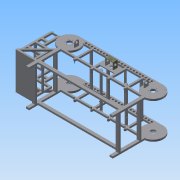
# Autodesk Inventor part: 整体支架
Saved by Autodesk Inventor 2015 (Build 190159000, 159)
## iProperties
Created: 2017-05-04
Part Number: 整体支架
Material: 常规
Document SubType Name: Modeling
Designer: Administrator
Density: 1 g/cm^3
Appearance: 默认
Author: Administrator
Autodesk Inventor part; units mm, degrees
ref_plane "YZ Plane" through (0, 0, 0) normal (1, 0, 0) x (0, 1, 0)
ref_plane "XZ Plane" through (0, 0, 0) normal (0, 1, 0) x (-1, 0, 0)
sketch "草图1" plane through (0, 0, 0) normal (0, 0, 1) x (1, 0, 0)
  circle A0 centre (0, 0) radius 141.3842
  line L0 (-50, 166.3842) -> (50, 166.3842)
  line L1 (50, 166.3842) -> (50, 141.3842)
  line L2 (50, 141.3842) -> (-50, 141.3842)
  line L3 (-50, 141.3842) -> (-50, 166.3842)
  line L4 (0, 0) -> (0, 76.7752)
  line L5 (0, 0) -> (71.7187, 0)
  line L6 (-57.3473, 163.9969) -> (-42.6527, 143.7715)
  line L7 (-42.6527, 143.7715) -> (-123.5544, 84.9929)
  line L8 (-123.5544, 84.9929) -> (-138.249, 105.2184)
  line L9 (-142.7899, 98.9684) -> (-119.0135, 91.2429)
  line L10 (-119.0135, 91.2429) -> (-149.9152, -3.8627)
  line L11 (-149.9152, -3.8627) -> (-173.6916, 3.8627)
  line L12 (-173.6916, -3.8627) -> (-149.9152, 3.8627)
  line L13 (-149.9152, 3.8627) -> (-119.0135, -91.2429)
  line L14 (-119.0135, -91.2429) -> (-142.7899, -98.9684)
  line L15 (-138.249, -105.2184) -> (-123.5544, -84.9929)
  line L16 (-123.5544, -84.9929) -> (-42.6527, -143.7715)
  line L17 (-42.6527, -143.7715) -> (-57.3473, -163.9969)
  line L18 (-50, -166.3842) -> (-50, -141.3842)
  line L19 (-50, -141.3842) -> (50, -141.3842)
  line L20 (50, -141.3842) -> (50, -166.3842)
  line L21 (-10, 166.3842) -> (-20, 141.3842)
  line L22 (10, 166.3842) -> (20, 141.3842)
  arc A1 (18.4913, 145.1558) -> (24.0622, 141.3842) centre (24.0622, 147.3842) ccw
  arc A2 (-24.0622, 141.3842) -> (-18.4913, 145.1558) centre (-24.0622, 147.3842) ccw
  arc A3 (-19.7673, 141.9659) -> (-40.4509, 137.5092) centre (0, 0) ccw
  circle A4 centre (150, 128.8842) radius 12.5
  circle A5 centre (150, 128.8842) radius 17.5
  line L23 (0, 168.8842) -> (1400, 168.8842)
  line L24 (1400, 168.8842) -> (1400, 101.3842)
  line L25 (1400, 101.3842) -> (0, 101.3842)
  line L26 (0, 101.3842) -> (0, 168.8842)
  circle A6 centre (200, 128.8842) radius 17.5
  circle A7 centre (250, 128.8842) radius 17.5
  circle A8 centre (300, 128.8842) radius 17.5
  circle A9 centre (350, 128.8842) radius 17.5
  circle A10 centre (400, 128.8842) radius 17.5
  circle A11 centre (450, 128.8842) radius 17.5
  circle A12 centre (500, 128.8842) radius 17.5
  circle A13 centre (550, 128.8842) radius 17.5
  circle A14 centre (600, 128.8842) radius 17.5
  circle A15 centre (650, 128.8842) radius 17.5
  circle A16 centre (700, 128.8842) radius 17.5
  circle A17 centre (750, 128.8842) radius 17.5
  circle A18 centre (800, 128.8842) radius 17.5
  circle A19 centre (850, 128.8842) radius 17.5
  circle A20 centre (900, 128.8842) radius 17.5
  circle A21 centre (950, 128.8842) radius 17.5
  circle A22 centre (1000, 128.8842) radius 17.5
  circle A23 centre (1050, 128.8842) radius 17.5
  circle A24 centre (1100, 128.8842) radius 17.5
  circle A25 centre (1150, 128.8842) radius 17.5
  circle A26 centre (1200, 128.8842) radius 17.5
  circle A27 centre (1250, 128.8842) radius 17.5
  line L27 (265, 101.3842) -> (295, 101.3842)
  line L28 (295, 101.3842) -> (295, -191.3842)
  line L29 (265, -191.3842) -> (265, 101.3842)
  arc A28 (280, -166.3842) -> (265, -171.3842) centre (280, -191.3842) ccw
  line L30 (0, -166.3842) -> (1400, -166.3842)
  line L31 (1400, -166.3842) -> (1400, -141.3842)
  line L32 (1400, -141.3842) -> (0, -141.3842)
  line L33 (0, -141.3842) -> (0, -166.3842)
  arc A29 (265, -191.3842) -> (295, -191.3842) centre (280, -191.3842) ccw
  line L34 (545, 101.3842) -> (575, 101.3842)
  line L35 (575, 101.3842) -> (575, -191.3842)
  line L36 (545, -191.3842) -> (545, 101.3842)
  arc A30 (545, -191.3842) -> (575, -191.3842) centre (560, -191.3842) ccw
  line L37 (825, 101.3842) -> (855, 101.3842)
  line L38 (855, 101.3842) -> (855, -191.3842)
  line L39 (825, -191.3842) -> (825, 101.3842)
  arc A31 (825, -191.3842) -> (855, -191.3842) centre (840, -191.3842) ccw
  line L40 (1105, 101.3842) -> (1135, 101.3842)
  line L41 (1135, 101.3842) -> (1135, -191.3842)
  line L42 (1105, -191.3842) -> (1105, 101.3842)
  arc A32 (1105, -191.3842) -> (1135, -191.3842) centre (1120, -191.3842) ccw
  point P0 (0, 166.3842)
  point P1 (-50, 153.8842)
  point P2 (545, -171.3842)
  point P3 (825, -171.3842)
  point P4 (1105, -171.3842)
  dimension "d0" = 76.7752
  dimension "d1" = 71.7187
  dimension "d2" = 25
  dimension "d3" = 100
  dimension "d6" = 180
  dimension "d8" = 20
  dimension "d9" = 40
  dimension "d11" = 12
  dimension "d12" = 12
  dimension "d13" = 20.6835
  dimension "d14" = 25
  dimension "d15" = 35
  dimension "d16" = 150
  dimension "d17" = 40
  dimension "d18" = 27.5
  dimension "d19" = 1400
  dimension "d22" = 50
  dimension "d27" = 30
  dimension "d28" = 265
  dimension "d29" = 50
  dimension "d32" = 1400
  dimension "d33" = 25
  dimension "d36" = 280
  constraints: 86 end point, 33 centre point, 17 point on line, 16 point on circle, 10 tangent, 7 horizontal, 7 parallel, 4 perpendicular, 3 coincident, 3 midpoint, 2 collinear, 2 concentric, 1 vertical, 111 other
  measures "d0" distance of L4.start L4.end
  measures "d1" distance of L4.start L5.end
  measures "d2" distance of L2.end L0.start
  measures "d3" distance of L0.start L0.end
  measures "d8" distance of L22.start L21.start
  measures "d9" distance of L22.end L21.end
  measures "d11" diameter of A1
  measures "d12" diameter of A2
  measures "d13" horizontal distance of A3.start A3.end
  measures "d14" diameter of A4
  measures "d15" diameter of A5
  measures "d16" distance from line of L4 A4.centre
  measures "d17" distance from line of L23 A5.centre
  measures "d18" distance from line of L25 A4.centre
  measures "d19" distance of L23.start L23.end
  measures "d22" distance of A5.centre A6.centre
  measures "d27" distance between parallel lines of L28 L29
  measures "d28" distance from line of point (0, 0) L29
  measures "d29" diameter of A28
  measures "d32" distance of L32.end L31.end
  measures "d33" distance of L32.end L30.start
  measures "d36" distance of L29.start L36.start
extrude "拉伸1" add sketch "草图1" against normal blind 30 contours L19 L20 L30 L33 | L32 L29 L30 L20 | L25 L26 A0 | A0 L2 L1 L0 L26 L23 L24 L25 | L32 L28 L30 L29 | L29 L25 L28 L32 | L26 L0 L22 L2 | L30 A28 L29 | L32 L36 L30 L28 | A28 L30 L28 A29 L29 | L36 L25 L35 L32 | L32 L35 L30 L36 | A1 L22 L0 L1 L2 | L30 L35 A30 L36 | L32 L39 L30 L35 | L39 L25 L38 L32 | L32 L38 L30 L39 | L30 L38 A31 L39 | L32 L42 L30 L38 | L41 L32 L42 L25 | L32 L41 L30 L42 | L32 L31 L30 L41 | L30 L41 A32 L42 picked at (61.7806, 104.7908)
sketch "草图2" plane through (0, 0, 0) normal (0, 0, 1) x (1, 0, 0)
  circle A0 centre (0, 0) radius 168.8842
  line L0 (1400, 168.8842) -> (0, 168.8842) projected
  line L1 (0, -166.3842) -> (1400, -166.3842)
  line L2 (1400, -166.3842) -> (1400, -168.8842)
  line L3 (1400, -168.8842) -> (0, -168.8842)
  line L4 (0, -168.8842) -> (0, -166.3842)
  circle A1 centre (1400, 0) radius 168.8842
  dimension "d45" = 1400
  constraints: 8 end point, 2 centre point, 2 horizontal, 2 parallel, 2 tangent, 1 coincident, 1 perpendicular, 2 other
  measures "d45" distance of A0.centre A1.centre
extrude "拉伸2" add sketch "草图2" against normal blind 30 contours A0 L1 L4 | L1 A1 L3 A0 | A0 L4 L1 | A1 L2 L1 | L1 L2 A1
sketch "草图5" plane through (0, 0, 0) normal (0, 0, 1) x (1, 0, 0)
  line L0 (-25, -167.0235) -> (25, -167.0235)
  line L1 (25, -167.0235) -> (25, -700)
  line L2 (25, -700) -> (-25, -700)
  line L3 (-25, -700) -> (-25, -167.0235)
  arc A0 (0, 168.8842) -> (0, -168.8842) centre (0, 0) ccw projected
  dimension "d67" = 700
  dimension "d68" = 50
  constraints: 8 end point, 2 parallel, 2 point on circle, 1 horizontal, 1 perpendicular
  measures "d67" distance from line of point (0, 0) L2
  measures "d68" distance of L1.end L2.end
extrude "拉伸5" add sketch "草图5" against normal blind 30
pattern_linear "矩形阵列2" count 2 spacing 1400 along (1, 0, 0) of "拉伸5"
sketch "草图6" plane through (0, 0, 0) normal (0, 0, 1) x (1, 0, 0)
  line L0 (25, -168.8842) -> (25, -700) projected
  line L1 (1375, -700) -> (1375, -168.8842) projected
  line L2 (25, -500) -> (1375, -500)
  line L3 (1375, -500) -> (1375, -550)
  line L4 (1375, -550) -> (25, -550)
  line L5 (25, -550) -> (25, -500)
  point P0 (0, 0)
  dimension "d74" = 500
  dimension "d75" = 50
  constraints: 8 end point, 2 parallel, 2 point on line, 1 horizontal, 1 perpendicular
  measures "d74" distance from line of point (0, 0) L2
  measures "d75" distance between parallel lines of L2 L4
extrude "拉伸6" add sketch "草图6" against normal blind 30
pattern_linear "矩形阵列14" count 2 spacing 590 along (0, 0, -1) of "拉伸1", "拉伸6", "拉伸5", "矩形阵列2", "拉伸2"
sketch "草图9" plane through (-25, -700, -590) normal (-1, 0, 0) x (0, 0, 1)
  line L0 (-30, 100) -> (590, 100)
  line L1 (590, 100) -> (590, 130)
  line L2 (590, 130) -> (-30, 130)
  line L3 (-30, 130) -> (-30, 100)
  line L4 (-30, 0) -> (-30, 532.9765) projected
  line L5 (590, 0) -> (590, 532.9765) projected
  line L6 (0, 0) -> (-30, 0) projected
  point P0 (590, 700)
  dimension "d138" = 30
  dimension "d139" = 100
  constraints: 8 end point, 2 collinear, 2 parallel, 1 horizontal, 1 perpendicular
  measures "d138" distance of L2.end L0.start
  measures "d139" distance between parallel lines of L6 L0
extrude "拉伸9" add sketch "草图9" against normal blind 50
pattern_linear "矩形阵列15" count 2 spacing 1400 along (1, 0, 0) of "拉伸9"
sketch "草图10" plane through (0, 0, 0) normal (0, 0, 1) x (1, 0, 0)
  line L0 (295, -141.3842) -> (295, 101.3842) projected
  line L1 (265, 101.3842) -> (295, 101.3842)
  line L2 (295, 101.3842) -> (295, 71.3842)
  line L3 (295, 71.3842) -> (265, 71.3842)
  line L4 (265, 71.3842) -> (265, 101.3842)
  point P0 (0, 0)
  dimension "d145" = 30
  constraints: 8 end point, 2 parallel, 1 horizontal, 1 perpendicular, 1 point on line
  measures "d145" distance between parallel lines of L1 L3
extrude "拉伸10" add sketch "草图10" against normal blind 590
pattern_linear "矩形阵列16" count 4 spacing 280 along (1, 0, 0) of "拉伸10"
pattern_linear "矩形阵列17" count 2 spacing 350 along (0, 1, 0) of "拉伸9", "矩形阵列15"
sketch "草图11" plane through (0, 0, 0) normal (0, 0, 1) x (1, 0, 0)
  circle A0 centre (1400, 0) radius 40
  arc A1 (1264.9329, 101.3842) -> (1307.6291, -141.3842) centre (1400, 0) ccw projected
  point P0 (0, 0)
  dimension "d154" = 80
  constraints: 1 centre point, 1 concentric
  measures "d154" diameter of A0
extrude "拉伸11" cut sketch "草图11" against normal blind 30
sketch "草图12" plane through (0, 0, 0) normal (0, 0, 1) x (1, 0, 0)
  circle A0 centre (1400, 55) radius 4
  circle A1 centre (1400, 0) radius 40
  circle A2 centre (1400, 0) radius 40 projected
  line L0 (1400, 0) -> (1400, 25)
  point P0 (0, 0)
  dimension "d157" = 80
  dimension "d158" = 25
  dimension "d159" = 55
  dimension "d160" = 8
  constraints: 2 centre point, 2 end point, 1 concentric, 1 point on line, 1 vertical
  measures "d157" diameter of A1
  measures "d158" distance of L0.start L0.end
  measures "d159" distance of A1.centre A0.centre
  measures "d160" diameter of A0
extrude "拉伸12" cut sketch "草图12" against normal blind 30 contours A0
thread "螺纹5" size "M8x1.25" class "6H" standard "ANSI Metric M Profile" full length
pattern_circular "环形阵列3" count 6 over 360 about axis through (1400, 0, 0) along (0, 0, -1) of "拉伸12"
sketch "草图13" plane through (0, 168.8842, -590) normal (0, 0, 1) x (1, 0, 0)
  circle A0 centre (1400, -168.8842) radius 40
  circle A1 centre (1400, -168.8842) radius 40 projected
  point P0 (0, -168.8842)
  dimension "d168" = 80
  constraints: 1 centre point, 1 concentric
  measures "d168" diameter of A0
extrude "拉伸13" cut sketch "草图13" against normal blind 18
sketch "草图14" plane through (1400, 0, -608) normal (0, 0, 1) x (1, 0, 0)
  circle A0 centre (0, 0) radius 31
  circle A1 centre (0, 0) radius 40 projected
  point P0 (-1400, 0)
  dimension "d171" = 62
  constraints: 1 centre point, 1 concentric
  measures "d171" diameter of A0
extrude "拉伸14" cut sketch "草图14" against normal blind 5 contours A0
sketch "草图15" plane through (1400, 0, -613) normal (0, 0, 1) x (1, 0, 0)
  circle A0 centre (0, 0) radius 20
  circle A1 centre (0, 0) radius 31 projected
  point P0 (-1400, 0)
  dimension "d174" = 40
  constraints: 1 centre point, 1 concentric
  measures "d174" diameter of A0
extrude "拉伸15" cut sketch "草图15" against normal through all contours A0
pattern_linear "矩形阵列18" count 2 spacing 1400 along (-1, 0, 0) of "拉伸11", "拉伸12", "环形阵列3", "拉伸13", "拉伸14", "拉伸15"
sketch "草图16" plane through (0, 0, 0) normal (0, 0, 1) x (1, 0, 0)
  circle A0 centre (127.5, 151.3842) radius 2
  circle A1 centre (127.5, 106.3842) radius 2
  circle A2 centre (150, 128.8842) radius 17.5 projected
  point P0 (0, 0)
  dimension "d180" = 4
  dimension "d181" = 4
  dimension "d182" = 22.5
  dimension "d183" = 22.5
  dimension "d184" = 22.5
  dimension "d185" = 22.5
  constraints: 2 centre point
  measures "d180" diameter of A0
  measures "d181" diameter of A1
  measures "d182" horizontal distance of A2.centre A0.centre
  measures "d183" horizontal distance of A2.centre A1.centre
  measures "d184" horizontal distance of A2.centre A0.centre
  measures "d185" horizontal distance of A2.centre A1.centre
extrude "拉伸16" cut sketch "草图16" against normal through all contours A0 | A1
thread "螺纹6" size "M4x0.7" class "6H" standard "ANSI Metric M Profile" full length
thread "螺纹7" size "M4x0.7" class "6H" standard "ANSI Metric M Profile" full length
thread "螺纹8" size "M4x0.7" class "6H" standard "ANSI Metric M Profile" full length
thread "螺纹9" size "M4x0.7" class "6H" standard "ANSI Metric M Profile" full length
pattern_linear "矩形阵列19" count 2 spacing 1145 along (1, 0, 0) of "拉伸16"
pattern_linear "矩形阵列20" count 2 spacing 197.5 along (1, 0, 0) of "拉伸16"
pattern_linear "矩形阵列21" count 6 spacing 150 along (1, 0, 0) of "矩形阵列20"
sketch "草图17" plane through (0, 0, -30) normal (0, 0, -1) x (-1, 0, 0)
  circle A0 centre (-280, -191.3842) radius 10
  arc A1 (-295, -191.3842) -> (-265, -191.3842) centre (-280, -191.3842) ccw projected
  point P0 (0, 0)
  dimension "d205" = 20
  constraints: 1 centre point, 1 concentric
  measures "d205" diameter of A0
extrude "拉伸17" add sketch "草图17" along normal blind 5
sketch "草图18" plane through (280, -191.3842, -35) normal (0, 0, -1) x (-1, 0, 0)
  circle A0 centre (0, 0) radius 5
  circle A1 centre (0, 0) radius 10 projected
  point P0 (280, 191.3842)
  dimension "d208" = 10
  constraints: 1 centre point, 1 concentric
  measures "d208" diameter of A0
extrude "拉伸18" add sketch "草图18" along normal blind 28 contours A0
thread "螺纹10" size "M10x1.5" class "6g" standard "ANSI Metric M Profile" length 10
chamfer "倒角1" distance 0.25 angle 45 1 edges at (285, -191.3842, -63)
ref_plane "工作平面1" through (0, 0, -310) normal (0, 0, -1) x (-1, 0, 0)
mirror "镜像1" about plane through (0, 0, -310) normal (0, 0, -1) of "拉伸17", "拉伸18", "倒角1"
pattern_linear "矩形阵列22" count 4 spacing 280 along (1, 0, 0) of "拉伸17", "拉伸18", "倒角1", "镜像1"
sketch "草图19" plane through (0, 0, 0) normal (0, 0, 1) x (1, 0, 0)
  circle A0 centre (1410, 152.6729) radius 2.5
  arc A1 (1422.9168, 151.274) -> (1410, 152.6729) centre (1400, 0) ccw
  circle A2 centre (1400, 0) radius 40 projected
  point P0 (0, 0)
  dimension "d219" = 5
  dimension "d220" = 153
  dimension "d221" = 10
  constraints: 2 centre point, 2 point on circle, 1 concentric
  measures "d219" diameter of A0
  measures "d220" radius of A1
  measures "d221" horizontal distance of A1.centre A0.centre
extrude "拉伸19" cut sketch "草图19" against normal through all contours A0
thread "螺纹11" size "M5x0.8" class "6H" standard "ANSI Metric M Profile" full length
thread "螺纹12" size "M5x0.8" class "6H" standard "ANSI Metric M Profile" full length
pattern_circular "环形阵列4" count 6 over 172.5 about axis through (1400, 0, 0) along (0, 0, -1) of "拉伸19"
sketch "草图20" plane through (0, 168.8842, 0) normal (0, 1, 0) x (1, 0, 0)
  circle A0 centre (1390, 11) radius 4
  line L0 (1400, 0) -> (0, 0) projected
  line L1 (1400, 0) -> (1400, 30) projected
  circle A1 centre (1390, 609) radius 4
  line L2 (0, 620) -> (1400, 620) projected
  line L3 (1400, 590) -> (1400, 620) projected
  dimension "d231" = 8
  dimension "d232" = 11
  dimension "d233" = 10
  dimension "d234" = 8
  dimension "d235" = 11
  dimension "d236" = 10
  constraints: 2 centre point
  measures "d231" diameter of A0
  measures "d232" distance from line of L0 A0.centre
  measures "d233" distance from line of L1 A0.centre
  measures "d234" diameter of A1
  measures "d235" distance from line of L2 A1.centre
  measures "d236" distance from line of L3 A1.centre
extrude "拉伸20" cut sketch "草图20" against normal blind 22
thread "螺纹13" size "M8x1.25" class "6H" standard "ANSI Metric M Profile" full length
thread "螺纹14" size "M8x1.25" class "6H" standard "ANSI Metric M Profile" full length
pattern_linear "矩形阵列23" count 5 spacing 220 along (-1, 0, 0) of "拉伸20"
sketch "草图21" plane through (0, 168.8842, 0) normal (0, 1, 0) x (1, 0, 0)
  circle A0 centre (20, 13) radius 4
  circle A1 centre (113.75, 13) radius 4
  circle A2 centre (207.5, 13) radius 4
  circle A3 centre (20, 607) radius 4
  line L0 (135.0671, 590) -> (135.0671, 620) projected
  line L1 (265, 590) -> (92.3709, 590) projected
  circle A4 centre (113.75, 607) radius 4
  line L2 (0, 590) -> (0, 620) projected
  line L3 (0, 620) -> (1400, 620) projected
  circle A5 centre (207.5, 607) radius 4
  line L4 (0, 0) -> (0, 30) projected
  line L5 (1400, 0) -> (0, 0) projected
  dimension "d246" = 8
  dimension "d247" = 8
  dimension "d248" = 8
  dimension "d249" = 8
  dimension "d252" = 8
  dimension "d253" = 20
  dimension "d254" = 13
  dimension "d255" = 13
  dimension "d256" = 113.75
  dimension "d257" = 8
  dimension "d258" = 13
  dimension "d259" = 207.5
  dimension "d260" = 20
  dimension "d261" = 13
  dimension "d262" = 113.75
  dimension "d263" = 207.5
  dimension "d264" = 13
  dimension "d265" = 13
  constraints: 6 centre point
  measures "d246" diameter of A0
  measures "d247" diameter of A1
  measures "d248" diameter of A2
  measures "d249" diameter of A3
  measures "d252" diameter of A4
  measures "d253" distance from line of L2 A3.centre
  measures "d254" distance from line of L3 A3.centre
  measures "d255" distance from line of L3 A4.centre
  measures "d256" distance from line of L2 A4.centre
  measures "d257" diameter of A5
  measures "d258" distance from line of A5.centre L3
  measures "d259" distance from line of L2 A5.centre
  measures "d260" distance from line of L4 A0.centre
  measures "d261" distance from line of L5 A0.centre
  measures "d262" distance from line of L4 A1.centre
  measures "d263" distance from line of L4 A2.centre
  measures "d264" distance from line of L5 A1.centre
  measures "d265" distance from line of L5 A2.centre
extrude "拉伸21" cut sketch "草图21" against normal blind 22
thread "螺纹15" size "M8x1.25" class "6H" standard "ANSI Metric M Profile" full length
thread "螺纹16" size "M8x1.25" class "6H" standard "ANSI Metric M Profile" full length
thread "螺纹17" size "M8x1.25" class "6H" standard "ANSI Metric M Profile" full length
thread "螺纹18" size "M8x1.25" class "6H" standard "ANSI Metric M Profile" full length
thread "螺纹19" size "M8x1.25" class "6H" standard "ANSI Metric M Profile" full length
thread "螺纹20" size "M8x1.25" class "6H" standard "ANSI Metric M Profile" full length
sketch "草图22" plane through (0, 0, 0) normal (0, 0, 1) x (1, 0, 0)
  line L0 (-25, -570) -> (-25, -250) projected
  line L1 (-25, -550) -> (-350, -550)
  line L2 (-350, -550) -> (-350, -520)
  line L3 (-350, -520) -> (-25, -520)
  line L4 (-25, -520) -> (-25, -550)
  line L5 (25, -500) -> (1375, -500) projected
  line L6 (1375, -550) -> (25, -550) projected
  point P0 (0, 0)
  dimension "d280" = 325
  dimension "d281" = 30
  constraints: 8 end point, 2 parallel, 1 collinear, 1 horizontal, 1 perpendicular, 1 point on line
  measures "d280" distance of L1.start L1.end
  measures "d281" distance of L1.end L2.end
extrude "拉伸22" add sketch "草图22" against normal up to surface (620 mm away)
sketch "草图23" plane through (0, 0, 0) normal (0, 0, 1) x (1, 0, 0)
  line L0 (-350, -520) -> (-25, -195)
  line L1 (-25, -520) -> (-25, -167.0235) projected
  line L2 (-307.5736, -520) -> (-25, -237.4264)
  line L3 (-25, -520) -> (-350, -520) projected
  line L4 (-350, -520) -> (-25, -520) projected
  line L5 (-350, -520) -> (-307.5736, -520)
  line L6 (-25, -195) -> (-25, -237.4264)
  point P0 (0, 0)
  dimension "d284" = 135
  dimension "d285" = 30
  constraints: 8 end point, 5 point on line, 1 collinear, 1 parallel
  measures "d284" angle of L3 L2
  measures "d285" distance between parallel lines of L0 L2
extrude "拉伸23" add sketch "草图23" against normal blind 30 contours L0 L1 L2 L3
pattern_linear "矩形阵列24" count 2 spacing 590 along (0, 0, -1) of "拉伸23"
sketch "草图25" plane through (0, 168.8842, -590) normal (0, 0, 1) x (1, 0, 0)
  line L0 (-350, -688.8842) -> (-70, -688.8842)
  line L1 (-70, -688.8842) -> (-70, -388.8842)
  line L2 (-70, -388.8842) -> (-350, -388.8842)
  line L3 (-350, -388.8842) -> (-350, -688.8842)
  line L4 (-200, -388.8842) -> (-350, -388.8842)
  line L5 (-350, -388.8842) -> (-350, -108.8842)
  line L6 (-350, -108.8842) -> (-200, -108.8842)
  line L7 (-200, -108.8842) -> (-200, -388.8842)
  line L8 (-320, -418.8842) -> (-100, -418.8842)
  line L9 (-100, -418.8842) -> (-100, -523.8842)
  line L10 (-100, -523.8842) -> (-320, -523.8842)
  line L11 (-320, -523.8842) -> (-320, -418.8842)
  line L12 (-320, -553.8842) -> (-100, -553.8842)
  line L13 (-100, -553.8842) -> (-100, -658.8842)
  line L14 (-100, -658.8842) -> (-320, -658.8842)
  line L15 (-320, -658.8842) -> (-320, -553.8842)
  line L16 (-320, -138.8842) -> (-230, -138.8842)
  line L17 (-230, -138.8842) -> (-230, -288.8842)
  line L18 (-230, -288.8842) -> (-320, -288.8842)
  line L19 (-320, -288.8842) -> (-320, -138.8842)
  line L20 (-320, -318.8842) -> (-230, -318.8842)
  line L21 (-230, -318.8842) -> (-230, -388.8842)
  line L22 (-230, -388.8842) -> (-320, -388.8842)
  line L23 (-320, -388.8842) -> (-320, -318.8842)
  point P0 (0, -168.8842)
  dimension "d291" = 280
  dimension "d292" = 300
  dimension "d293" = 150
  dimension "d294" = 280
  dimension "d295" = 30
  dimension "d296" = 30
  dimension "d297" = 30
  dimension "d298" = 30
  dimension "d299" = 30
  dimension "d300" = 30
  dimension "d301" = 30
  dimension "d302" = 30
  dimension "d303" = 30
  dimension "d304" = 150
  dimension "d305" = 105
  constraints: 48 end point, 12 parallel, 6 horizontal, 6 perpendicular, 5 point on line, 2 collinear
  measures "d291" distance of L2.end L1.end
  measures "d292" distance of L2.end L0.start
  measures "d293" distance of L5.end L6.end
  measures "d294" distance of L4.end L5.end
  measures "d295" distance between parallel lines of L3 L11
  measures "d296" distance between parallel lines of L9 L1
  measures "d297" distance between parallel lines of L2 L8
  measures "d298" distance between parallel lines of L12 L10
  measures "d299" distance between parallel lines of L0 L14
  measures "d300" distance between parallel lines of L20 L18
  measures "d301" distance between parallel lines of L7 L21
  measures "d302" distance between parallel lines of L5 L23
  measures "d303" distance between parallel lines of L6 L16
  measures "d304" distance between parallel lines of L16 L18
  measures "d305" distance between parallel lines of L14 L12
extrude "拉伸24" add sketch "草图25" along normal blind 30 contours L3 L2 L1 L0 | L5 L6 L7 L2 L21 L20 L23
pattern_linear "矩形阵列25" count 2 spacing 530 along (0, 0, 1) of "拉伸24"
sketch "草图26" plane through (-350, -550, -620) normal (-1, 0, 0) x (0, 0, 1)
  line L0 (30, 300) -> (30, -20) projected
  line L1 (590, 50) -> (590, 300) projected
  line L2 (30, 300) -> (590, 300)
  line L3 (590, 300) -> (590, 330)
  line L4 (590, 330) -> (30, 330)
  line L5 (30, 330) -> (30, 300)
  line L6 (30, 330) -> (60, 330) projected
  line L7 (30, 300) -> (60, 300) projected
  point P0 (620, 550)
  constraints: 8 end point, 2 collinear, 2 parallel, 2 point on line, 1 horizontal, 1 perpendicular
extrude "拉伸25" add sketch "草图26" against normal blind 30
sketch "草图27" plane through (0, 168.8842, -560) normal (0, 0, 1) x (1, 0, 0)
  line L0 (-85, -523.8842) -> (-70, -523.8842)
  line L1 (-70, -523.8842) -> (-70, -553.8842)
  line L2 (-70, -553.8842) -> (-85, -553.8842)
  line L3 (-85, -553.8842) -> (-85, -523.8842)
  line L4 (-70, -688.8842) -> (-70, -388.8842) projected
  line L5 (-320, -553.8842) -> (-100, -553.8842) projected
  line L6 (-100, -523.8842) -> (-320, -523.8842) projected
  point P0 (0, -168.8842)
  dimension "d313" = 15
  constraints: 8 end point, 3 collinear, 2 parallel, 1 horizontal, 1 perpendicular
  measures "d313" distance of L1.end L2.end
extrude "拉伸26" add sketch "草图27" along normal up to next
sketch "草图28" plane through (-85, -385, -560) normal (-1, 0, 0) x (0, 0, 1)
  line L0 (0, 0) -> (0, 30) projected
  line L1 (0, 15) -> (10, 15)
  line L2 (10, 15) -> (10, 0)
  line L3 (10, 0) -> (0, 0)
  line L4 (0, 0) -> (0, 15)
  line L5 (500, 0) -> (490, 0)
  line L6 (490, 0) -> (490, 15)
  line L7 (490, 15) -> (500, 15)
  line L8 (500, 15) -> (500, 0)
  point P0 (560, 385)
  dimension "d316" = 15
  dimension "d317" = 10
  dimension "d318" = 10
  constraints: 16 end point, 4 parallel, 2 horizontal, 2 perpendicular, 1 midpoint, 1 point on line
  measures "d316" distance of L1.end L2.end
  measures "d317" distance of L1.start L1.end
  measures "d318" distance of L6.end L7.end
extrude "拉伸27" add sketch "草图28" along normal up to surface (265 mm away)
sketch "草图29" plane through (0, 168.8842, -560) normal (0, 0, 1) x (1, 0, 0)
  line L0 (-70, -688.8842) -> (-85, -688.8842)
  line L1 (-85, -688.8842) -> (-85, -658.8842)
  line L2 (-85, -658.8842) -> (-70, -658.8842)
  line L3 (-70, -658.8842) -> (-70, -688.8842)
  line L4 (-100, -658.8842) -> (-320, -658.8842) projected
  point P0 (0, -168.8842)
  dimension "d321" = 15
  constraints: 8 end point, 2 parallel, 1 collinear, 1 horizontal, 1 perpendicular
  measures "d321" distance of L1.end L2.end
extrude "拉伸28" add sketch "草图29" along normal up to next
sketch "草图30" plane through (-85, -385, -550) normal (0, 0, 1) x (1, 0, 0)
  line L0 (-265, 15) -> (0, 15) projected
  circle A0 centre (-260, 15) radius 5
  line L1 (-265, 15) -> (-265, 0) projected
  point P0 (85, 385)
  dimension "d324" = 10
  constraints: 1 centre point, 1 point on line, 1 tangent
  measures "d324" diameter of A0
extrude "拉伸29" add sketch "草图30" against normal blind 10
pattern_linear "矩形阵列26" count 2 spacing 490 along (0, 0, 1) of "拉伸29"
pattern_linear "矩形阵列27" count 2 spacing 150 along (0, -1, 0) of "拉伸29", "矩形阵列26"
sketch "草图31" plane through (-350, -220, -60) normal (0, 1, 0) x (1, 0, 0)
  line L0 (30, 500) -> (30, 0) projected
  line L1 (30, 340) -> (150, 340)
  line L2 (150, 340) -> (150, 160)
  line L3 (150, 160) -> (30, 160)
  line L4 (30, 160) -> (30, 340)
  line L5 (120, 310) -> (30, 310)
  line L6 (30, 310) -> (30, 190)
  line L7 (30, 190) -> (120, 190)
  line L8 (120, 190) -> (120, 310)
  point P0 (350, -60)
  point P1 (30, 250)
  dimension "d333" = 120
  dimension "d334" = 180
  dimension "d335" = 30
  dimension "d336" = 30
  dimension "d337" = 30
  constraints: 16 end point, 4 parallel, 2 horizontal, 2 midpoint, 2 perpendicular, 2 point on line
  measures "d333" distance of L2.end L3.end
  measures "d334" distance of L1.end L2.end
  measures "d335" distance between parallel lines of L2 L8
  measures "d336" distance between parallel lines of L3 L7
  measures "d337" distance between parallel lines of L1 L5
extrude "拉伸30" add sketch "草图31" against normal blind 30 contours L1 L2 L3 L0 L7 L8 L5
sketch "草图32" plane through (-350, -220, -60) normal (0, 1, 0) x (1, 0, 0)
  line L0 (135, 325) -> (30, 325)
  line L1 (30, 325) -> (30, 175)
  line L2 (30, 175) -> (135, 175)
  line L3 (135, 175) -> (135, 325)
  line L4 (30, 310) -> (30, 190) projected
  line L5 (150, 160) -> (150, 340) projected
  line L6 (30, 160) -> (150, 160) projected
  line L7 (150, 340) -> (30, 340) projected
  line L8 (30, 325) -> (15, 325)
  line L9 (375, -30) -> (375, 530) projected
  line L10 (15, 325) -> (15, 175)
  line L11 (15, 175) -> (30, 175)
  point P0 (350, -60)
  dimension "d340" = 15
  dimension "d341" = 15
  dimension "d342" = 15
  dimension "d343" = 15
  constraints: 14 end point, 4 perpendicular, 2 parallel, 1 collinear, 1 horizontal
  measures "d340" distance between parallel lines of L5 L3
  measures "d341" distance between parallel lines of L6 L2
  measures "d342" distance between parallel lines of L7 L0
  measures "d343" distance of L0.end L8.end
extrude "拉伸31" cut sketch "草图32" against normal blind 10
sketch "草图34" plane through (-350, 60, -590) normal (0, 1, 0) x (1, 0, 0)
  line L0 (150, 0) -> (0, 0)
  line L1 (0, 0) -> (0, -30)
  line L2 (0, -30) -> (150, -30)
  line L3 (150, -30) -> (150, 0)
  line L4 (150, -530) -> (0, -530)
  line L5 (0, -530) -> (0, -560)
  line L6 (0, -560) -> (150, -560)
  line L7 (150, -560) -> (150, -530)
  circle A0 centre (135, -15) radius 5
  circle A1 centre (15, -15) radius 5
  circle A2 centre (135, -545) radius 5
  circle A3 centre (15, -545) radius 5
  point P0 (350, -590)
  dimension "d360" = 30
  dimension "d361" = 10
  dimension "d362" = 10
  dimension "d363" = 10
  dimension "d364" = 10
  dimension "d365" = 15
  dimension "d366" = 15
  dimension "d367" = 15
  dimension "d368" = 15
  dimension "d369" = 15
  dimension "d370" = 15
  dimension "d371" = 15
  dimension "d372" = 15
  constraints: 16 end point, 4 centre point, 4 parallel, 2 horizontal, 2 perpendicular, 1 point on line
  measures "d360" distance of L6.end L4.start
  measures "d361" diameter of A0
  measures "d362" diameter of A1
  measures "d363" diameter of A2
  measures "d364" diameter of A3
  measures "d365" distance from line of L3 A0.centre
  measures "d366" distance from line of L2 A0.centre
  measures "d367" distance from line of L2 A1.centre
  measures "d368" distance from line of L1 A1.centre
  measures "d369" distance from line of L5 A3.centre
  measures "d370" distance from line of L6 A3.centre
  measures "d371" distance from line of A2.centre L6
  measures "d372" distance from line of L7 A2.centre
extrude "拉伸33" cut sketch "草图34" against normal blind 20
thread "螺纹21" size "M10x1.5" class "6g" standard "ANSI Metric M Profile" length 10
thread "螺纹22" size "M10x1.5" class "6g" standard "ANSI Metric M Profile" length 10
thread "螺纹23" size "M10x1.5" class "6g" standard "ANSI Metric M Profile" length 10
thread "螺纹24" size "M10x1.5" class "6g" standard "ANSI Metric M Profile" length 10
chamfer "倒角2" distance 0.5 angle 45 4 edges at (-340, 60, -575) (-220, 60, -575) (-220, 60, -45) (-340, 60, -45)
sketch "草图35" plane through (0, 0, 0) normal (0, 0, 1) x (1, 0, 0)
  line L0 (110, 35) -> (124, 35)
  line L1 (124, 35) -> (124, -35)
  line L2 (124, -35) -> (110, -35)
  line L3 (110, -35) -> (110, 35)
  line L4 (0, 0) -> (110, 0)
  dimension "d386" = 70
  dimension "d387" = 14
  dimension "d388" = 110
  constraints: 10 end point, 2 horizontal, 2 parallel, 1 midpoint, 1 perpendicular
  measures "d386" distance of L0.end L1.end
  measures "d387" distance of L0.start L0.end
  measures "d388" distance of L4.start L4.end
extrude "拉伸34" add sketch "草图35" along normal blind 99.418
fillet "圆角2" radius 35 2 edges at (117, 35, 99.418) (117, -35, 99.418)
sketch "草图36" plane through (124, -35, 0) normal (1, 0, 0) x (0, 0, -1)
  circle A0 centre (-64.418, 35) radius 21
  arc A1 (-64.418, 70) -> (-64.418, 0) centre (-64.418, 35) ccw projected
  point P0 (0, 35)
  dimension "d392" = 42
  constraints: 1 centre point, 1 concentric
  measures "d392" diameter of A0
extrude "拉伸35" cut sketch "草图36" against normal through all
pattern_linear "矩形阵列28" count 2 spacing 1166 along (1, 0, 0) of "拉伸35", "拉伸34", "圆角2"
sketch "草图37" plane through (0, 0, 0) normal (0, 0, 1) x (1, 0, 0)
  line L0 (575, 70) -> (825, 70)
  line L1 (825, 70) -> (825, -70)
  line L2 (825, -70) -> (575, -70)
  line L3 (575, -70) -> (575, 70)
  line L4 (825, -141.3842) -> (825, 101.3842) projected
  line L5 (575, 101.3842) -> (575, -141.3842) projected
  point P0 (0, 0)
  dimension "d398" = 140
  dimension "d399" = 70
  constraints: 8 end point, 2 collinear, 2 parallel, 1 horizontal, 1 perpendicular
  measures "d398" distance of L2.end L0.start
  measures "d399" distance from line of point (0, 0) L2
extrude "拉伸36" add sketch "草图37" against normal blind 14
sketch "草图38" plane through (0, 0, 0) normal (0, 0, 1) x (1, 0, 0)
  line L0 (630, 35) -> (770, 35)
  line L1 (770, 35) -> (770, -35)
  line L2 (770, -35) -> (630, -35)
  line L3 (630, -35) -> (630, 35)
  point P0 (0, 0)
  dimension "d402" = 630
  dimension "d403" = 140
  dimension "d404" = 70
  dimension "d405" = 35
  constraints: 8 end point, 2 parallel, 1 horizontal, 1 perpendicular
  measures "d402" distance from line of point (0, 0) L3
  measures "d403" distance of L1.end L2.end
  measures "d404" distance of L0.end L1.end
  measures "d405" distance from line of point (0, 0) L2
extrude "拉伸37" add sketch "草图38" along normal blind 116.414
sketch "草图39" plane through (630, 35, 0) normal (0, 1, 0) x (1, 0, 0)
  line L0 (14, 0) -> (126, 0)
  line L1 (126, 0) -> (126, -102.414)
  line L2 (126, -102.414) -> (14, -102.414)
  line L3 (14, -102.414) -> (14, 0)
  line L4 (140, 0) -> (140, -116.414) projected
  line L5 (140, -116.414) -> (0, -116.414) projected
  line L6 (0, 0) -> (0, -116.414) projected
  line L7 (770, 0) -> (-630, 0) projected
  dimension "d408" = 14
  dimension "d409" = 14
  dimension "d410" = 14
  constraints: 8 end point, 2 parallel, 1 collinear, 1 horizontal, 1 perpendicular
  measures "d408" distance between parallel lines of L4 L1
  measures "d409" distance between parallel lines of L5 L2
  measures "d410" distance between parallel lines of L6 L3
extrude "拉伸38" cut sketch "草图39" against normal blind 70 contours L0 L1 L2 L3
sketch "草图40" plane through (630, -35, 0) normal (-1, 0, 0) x (0, 0, 1)
  circle A0 centre (64.418, 35) radius 21
  circle A1 centre (64.418, 35) radius 21 projected
  point P0 (0, 35)
  constraints: 2 concentric, 1 centre point
extrude "拉伸39" cut sketch "草图40" against normal blind 140
sketch "草图41" plane through (0, 0, -14) normal (0, 0, -1) x (-1, 0, 0)
  circle A0 centre (-700, 0) radius 21
  point P0 (0, 0)
  dimension "d415" = 42
  dimension "d416" = 700
  dimension "d417" = 0
  constraints: 1 centre point
  measures "d415" diameter of A0
  measures "d416" distance of point (0, 0) A0.centre
  measures "d417" vertical distance of point (0, 0) A0.centre
extrude "拉伸40" cut sketch "草图41" against normal blind 14
sketch "草图42" plane through (756, 35, 102.414) normal (0, 0, -1) x (-1, 0, 0)
  circle A0 centre (56, -35) radius 13.5
  circle A1 centre (56, -35) radius 21 projected
  point P0 (756, -35)
  dimension "d420" = 27
  constraints: 1 centre point, 1 concentric
  measures "d420" diameter of A0
extrude "拉伸41" add sketch "草图42" along normal blind 5 contours A0
sketch "草图43" plane through (700, 0, 97.414) normal (0, 0, -1) x (-1, 0, 0)
  circle A0 centre (0, 0) radius 10
  circle A1 centre (0, 0) radius 13.5 projected
  point P0 (700, 0)
  dimension "d423" = 20
  constraints: 1 centre point, 1 concentric
  measures "d423" diameter of A0
extrude "拉伸42" add sketch "草图43" along normal blind 18.378 contours A0
chamfer "倒角3" distance 0.5 angle 45 1 edges at (710, 0, 79.036)
sketch "草图44" plane through (0, 0, 0) normal (0, 1, 0) x (-1, 0, 0)
  line L0 (-709.175, 83.036) -> (-714.3537, 83.036)
  line L1 (-714.3537, 83.036) -> (-714.3537, 84.236)
  line L2 (-714.3537, 84.236) -> (-709.175, 84.236)
  line L3 (-709.175, 84.236) -> (-709.175, 83.036)
  line L4 (-690.5, 79.036) -> (-709.5, 79.036) projected
  line L5 (-630, 0) -> (-630, 116.414) projected
  line L6 (-700, 263.6968) -> (-700, -767.2828) projected
  point P0 (0, 0)
  dimension "d429" = 1.2
  dimension "d430" = 4
  dimension "d431" = 79.175
  dimension "d432" = 5.1787
  constraints: 8 end point, 2 parallel, 1 horizontal, 1 perpendicular
  measures "d429" distance of L0.end L1.end
  measures "d430" distance between parallel lines of L4 L0
  measures "d431" distance between parallel lines of L5 L3
  measures "d432" distance of L1.end L2.end
revolve "旋转1" cut sketch "草图44" angle 360 about axis through (700, 0, 97.414) along (0, 0, -1)
sketch "草图45" plane through (1400, 168.8842, -620) normal (0, 0, -1) x (-1, 0, 0)
  line L0 (295, -310.2684) -> (545, -310.2684) projected
  line L1 (335, -310.2684) -> (315, -310.2684)
  line L2 (315, -310.2684) -> (315, -280.2684)
  line L3 (315, -280.2684) -> (335, -280.2684)
  line L4 (335, -280.2684) -> (335, -310.2684)
  line L5 (755, -310.2684) -> (735, -310.2684)
  line L6 (735, -310.2684) -> (735, -280.2684)
  line L7 (735, -280.2684) -> (755, -280.2684)
  line L8 (755, -280.2684) -> (755, -310.2684)
  arc A0 (335, -280.2684) -> (315, -280.2684) centre (325, -280.2684) ccw
  arc A1 (755, -280.2684) -> (735, -280.2684) centre (745, -280.2684) ccw
  line L9 (545, -337.7684) -> (545, -360.2684) projected
  line L10 (575, -360.2684) -> (575, -337.7684) projected
  point P0 (1400, -168.8842)
  dimension "d434" = 20
  dimension "d435" = 20
  dimension "d436" = 30
  dimension "d437" = 30
  dimension "d438" = 210
  dimension "d439" = 160
  constraints: 16 end point, 4 parallel, 4 point on circle, 4 tangent, 2 centre point, 2 horizontal, 2 perpendicular, 2 point on line
  measures "d434" distance of L2.end L3.end
  measures "d435" distance of L6.end L7.end
  measures "d436" distance of L1.end L2.end
  measures "d437" distance of L7.end L5.start
  measures "d438" distance between parallel lines of L9 L4
  measures "d439" distance between parallel lines of L6 L10
extrude "拉伸43" add sketch "草图45" against normal up to surface (620 mm away)
sketch "草图46" plane through (1400, 168.8842, -620) normal (0, 0, -1) x (-1, 0, 0)
  line L0 (545, -67.5) -> (545, -310.2684) projected
  line L1 (545, -80.2684) -> (575, -80.2684)
  line L2 (575, -80.2684) -> (575, -310.2684)
  line L3 (575, -310.2684) -> (545, -310.2684)
  line L4 (545, -310.2684) -> (545, -80.2684)
  point P0 (1400, -168.8842)
  dimension "d442" = 230
  constraints: 8 end point, 2 parallel, 1 horizontal, 1 perpendicular, 1 point on line
  measures "d442" distance of L1.end L2.end
extrude "拉伸44" cut sketch "草图46" against normal up to surface (590 mm away)
sketch "草图47" plane through (1400, 168.8842, -620) normal (0, 0, -1) x (-1, 0, 0)
  line L0 (825, -67.5) -> (825, -310.2684) projected
  line L1 (295, -67.5) -> (825, -67.5)
  line L2 (825, -67.5) -> (825, -80.2684)
  line L3 (825, -80.2684) -> (295, -80.2684)
  line L4 (295, -80.2684) -> (295, -67.5)
  line L5 (545, -80.2684) -> (575, -80.2684) projected
  point P0 (1400, -168.8842)
  constraints: 8 end point, 2 parallel, 1 collinear, 1 horizontal, 1 perpendicular, 1 point on line
extrude "拉伸45" add sketch "草图47" against normal blind 30
sketch "草图48" plane through (0, 0, 0) normal (0, 0, 1) x (1, 0, 0)
  circle A0 centre (655, -111.3842) radius 10
  arc A1 (665, -111.3842) -> (645, -111.3842) centre (655, -111.3842) ccw projected
  line L0 (646.4615, -106.179) -> (625, -141.3842)
  line L1 (575, -141.3842) -> (645, -141.3842) projected
  line L2 (663.5385, -106.179) -> (685, -141.3842)
  line L3 (685, -141.3842) -> (625, -141.3842)
  circle A2 centre (1075, -111.3842) radius 10
  line L4 (1066.4615, -106.179) -> (1045, -141.3842)
  line L5 (1083.5385, -106.179) -> (1105, -141.3842)
  line L6 (1105, -141.3842) -> (1045, -141.3842)
  line L7 (665, -141.3842) -> (1065, -141.3842) projected
  line L8 (1105, -141.3842) -> (1085, -141.3842) projected
  arc A3 (1085, -111.3842) -> (1065, -111.3842) centre (1075, -111.3842) ccw projected
  point P0 (0, 0)
  dimension "d447" = 60
  dimension "d448" = 60
  constraints: 13 end point, 6 point on circle, 6 tangent, 2 centre point, 2 collinear, 2 concentric, 2 equal length, 2 point on line
  measures "d447" distance of L2.end L0.end
  measures "d448" distance of L5.end L4.end
extrude "拉伸46" add sketch "草图48" against normal blind 30 contours A0 L2 L3 L1 L0 | A2 L5 L6 L4
pattern_linear "矩形阵列29" count 2 spacing 590 along (0, 0, -1) of "拉伸46"
sketch "草图49" plane through (1085, -141.3842, -590) normal (1, 0, 0) x (0, 0, -1)
  circle A0 centre (-540, 15) radius 5
  line L0 (0, 0) -> (-560, 0) projected
  line L1 (-560, -25.6394) -> (-560, 310.2684) projected
  circle A1 centre (-110.5, 15) radius 5
  point P0 (-590, 141.3842)
  dimension "d454" = 10
  dimension "d455" = 15
  dimension "d456" = 20
  dimension "d457" = 10
  dimension "d458" = 15
  dimension "d459" = 429.5
  constraints: 2 centre point
  measures "d454" diameter of A0
  measures "d455" distance from line of L0 A0.centre
  measures "d456" distance from line of L1 A0.centre
  measures "d457" diameter of A1
  measures "d458" distance from line of L0 A1.centre
  measures "d459" distance of A0.centre A1.centre
extrude "拉伸47" add sketch "草图49" along normal blind 20
thread "螺纹25" size "M10x1.5" class "6g" standard "ANSI Metric M Profile" length 10
thread "螺纹26" size "M10x1.5" class "6g" standard "ANSI Metric M Profile" length 10
chamfer "倒角4" distance 1 angle 45 2 edges at (1105, -126.3842, -45) (1105, -126.3842, -474.5)
sketch "草图50" plane through (645, -141.3842, -590) normal (-1, 0, 0) x (0, 0, 1)
  circle A0 centre (540, 15) radius 5
  circle A1 centre (110.5, 15) radius 5
  line L0 (0, 0) -> (560, 0) projected
  line L1 (560, 181.3842) -> (560, -378.6158) projected
  point P0 (590, 141.3842)
  dimension "d469" = 10
  dimension "d470" = 10
  dimension "d471" = 15
  dimension "d472" = 20
  dimension "d473" = 15
  dimension "d474" = 429.5
  constraints: 2 centre point
  measures "d469" diameter of A0
  measures "d470" diameter of A1
  measures "d471" distance from line of L0 A0.centre
  measures "d472" distance from line of A0.centre L1
  measures "d473" distance from line of L0 A1.centre
  measures "d474" distance of A0.centre A1.centre
extrude "拉伸48" add sketch "草图50" along normal blind 20
thread "螺纹27" size "M10x1.5" class "6g" standard "ANSI Metric M Profile" length 10
thread "螺纹28" size "M10x1.5" class "6g" standard "ANSI Metric M Profile" length 10
chamfer "倒角5" distance 1 angle 45 2 edges at (625, -126.3842, -55) (625, -126.3842, -484.5)
equation "\"d393\" = d392"
